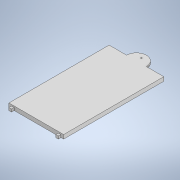
# Autodesk Inventor part: tapa pila
Saved by Autodesk Inventor 2020 (Build 240168000, 168)
## iProperties
Created: 2022-05-31
Part Number: tapa pila
Material: Generic
Document SubType Name: Modeling
Designer: juanc
Density: 1 g/cm^3
Appearance: Default
Author: juanc
Autodesk Inventor part; units mm, degrees
ref_plane "YZ Plane" through (0, 0, 0) normal (1, 0, 0) x (0, 1, 0)
ref_plane "XZ Plane" through (0, 0, 0) normal (0, 1, 0) x (-1, 0, 0)
ref_plane "XY Plane" through (0, 0, 0) normal (0, 0, 1) x (1, 0, 0)
sketch "Sketch1" plane through (0, 0, 0) normal (0, 1, 0) x (-1, 0, 0)
  line L0 (0, 0) -> (41.5, 0)
  line L1 (41.5, 0) -> (41.5, -76)
  line L2 (41.5, -76) -> (0, -76)
  line L3 (0, -76) -> (0, 0)
  dimension "d0" = 41.5
  dimension "d1" = 76
  constraints: 8 end point, 2 parallel, 1 horizontal, 1 perpendicular
  measures "d0" distance of L1.end L2.end
  measures "d1" distance of L0.end L1.end
extrude "Extrusion1" add sketch "Sketch1" along normal blind 3
sketch "Sketch2" plane through (-41.5, 0, 0) normal (0, 0, 1) x (1, 0, 0)
  line L0 (41.5, 0) -> (0, 0) construction
  line L1 (0, 0) -> (2, 0) construction
  line L2 (41.5, 0) -> (41.5, 3) construction
  line L3 (41.5, 0) -> (39.5, 0) construction
  line L4 (2, 0) -> (4, 0)
  line L5 (4, 0) -> (4, 2)
  line L6 (4, 2) -> (2, 2)
  line L7 (2, 2) -> (2, 0)
  line L8 (39.5, 0) -> (37.5, 0)
  line L9 (37.5, 0) -> (37.5, 2)
  line L10 (37.5, 2) -> (39.5, 2)
  line L11 (39.5, 2) -> (39.5, 0)
  dimension "d4" = 2
  dimension "d5" = 2
  dimension "d6" = 2
  dimension "d7" = 2
  dimension "d8" = 2
  dimension "d9" = 2
  constraints: 20 end point, 4 parallel, 2 horizontal, 2 perpendicular, 2 point on line
  measures "d4" distance of L0.end L1.end
  measures "d5" distance of L0.start L3.end
  measures "d6" distance of L6.end L5.end
  measures "d7" distance of L5.end L4.end
  measures "d8" distance of L9.end L10.end
  measures "d9" distance of L8.end L9.end
extrude "Extrusion2" add sketch "Sketch2" along normal blind 2
sketch "Sketch3" plane through (0, 3, 0) normal (0, 1, 0) x (1, 0, 0)
  line L0 (0, 76) -> (-41.5, 76) projected
  circle A0 centre (-20.75, 76) radius 7.5
  point P0 (0, 0)
  point P1 (-28.25, 76)
  point P2 (-13.25, 76)
  dimension "d12" = 15
  constraints: 1 centre point, 1 midpoint
  measures "d12" diameter of A0
extrude "Extrusion3" add sketch "Sketch3" against normal blind 1.5 contours L0 A0 picked at (-18.3226, 76.5983)
sketch "Sketch4" plane through (0, 3, 0) normal (0, 1, 0) x (1, 0, 0)
  line L0 (-28.25, 76) -> (-13.25, 76) construction
  line L1 (-20.75, 76) -> (-20.75, 79.75) construction
  point P0 (0, 0)
  dimension "d15" = 3.75
  constraints: 2 end point, 1 coincident, 1 midpoint, 1 vertical
  measures "d15" distance of L1.start L1.end
hole "Hole1" at (-20.75, 3, -79.75) direction (0, -1, 0) diameter 1 depth 2 tip angle 118
sketch "Sketch5" plane through (0, 0, 0) normal (0, -1, 0) x (1, 0, 0)
  line L0 (-28.25, -76) -> (-13.25, -76) construction
  line L1 (-20.75, -76) -> (-20.75, 0) construction
  line L2 (-41.5, 0) -> (0, 0) construction
  line L3 (-41.5, -76) -> (-41.5, 0) construction
  line L4 (-41.5, -76) -> (-20.75, 0) construction
  line L5 (-41.5, 0) -> (-20.75, -76) construction
  line L6 (-28.25, -76) -> (-41.5, -76) construction
  line L7 (-31.125, -76) -> (-31.125, -73) construction
  line L8 (-31.125, 0) -> (-31.125, -3) construction
  line L9 (-31.125, -73) -> (-31.125, -3) construction
  line L10 (-22.625, -64.5) -> (-22.625, -11.5)
  line L11 (-39.625, -11.5) -> (-39.625, -64.5)
  arc A0 (-39.625, -64.5) -> (-22.625, -64.5) centre (-31.125, -64.5) ccw
  arc A1 (-22.625, -11.5) -> (-39.625, -11.5) centre (-31.125, -11.5) ccw
  line L12 (-18.875, -64.5) -> (-18.875, -11.5)
  line L13 (-1.875, -11.5) -> (-1.875, -64.5)
  arc A2 (-18.875, -64.5) -> (-1.875, -64.5) centre (-10.375, -64.5) ccw
  arc A3 (-1.875, -11.5) -> (-18.875, -11.5) centre (-10.375, -11.5) ccw
  point P0 (-31.125, -38)
  dimension "d23" = 3
  dimension "d24" = 3
  dimension "d25" = 17
  constraints: 22 end point, 10 point on circle, 6 symmetric about line, 4 centre point, 4 point on line, 4 tangent, 3 midpoint, 3 vertical, 1 parallel, 2 other
  measures "d23" distance of L7.start L7.end
  measures "d24" distance of L8.start L8.end
  measures "d25" diameter of A1
extrude "Extrusion4" cut sketch "Sketch5" against normal blind 0.5
fillet "Fillet1" radius 2.5 8 edges at (-31.125, 0, -73) (-39.625, 0, -38) (-31.125, 0, -3) (-22.625, 0, -38) (-10.375, 0, -3) (-1.875, 0, -38) (-10.375, 0, -73) (-18.875, 0, -38)
body "Solid1"
